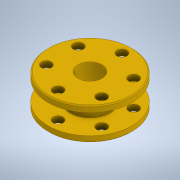
# Autodesk Inventor part: connecting rod hub
Saved by Autodesk Inventor 2020 (Build 240168000, 168)
## iProperties
Created: 2020-08-04
Part Number: connecting rod hub
Material: Generic
Document SubType Name: Modeling
Designer: benny
Density: 1 g/cm^3
Appearance: Gold
Author: benny
Autodesk Inventor part; units mm, degrees
ref_plane "YZ Plane" through (0, 0, 0) normal (1, 0, 0) x (0, 1, 0)
ref_plane "XZ Plane" through (0, 0, 0) normal (0, 1, 0) x (-1, 0, 0)
ref_plane "XY Plane" through (0, 0, 0) normal (0, 0, 1) x (1, 0, 0)
sketch "Sketch1" plane through (0, 0, 0) normal (0, 1, 0) x (-1, 0, 0)
  circle A0 centre (0, 0) radius 10
  dimension "d0" = 20
  constraints: 1 centre point, 1 coincident
  measures "d0" diameter of A0
extrude "Extrusion1" add sketch "Sketch1" along normal mid plane 10
sketch "Sketch2" plane through (0, 5, 0) normal (0, 1, 0) x (1, 0, 0)
  circle A0 centre (0, 0) radius 21
  dimension "d3" = 42
  constraints: 1 centre point, 1 coincident
  measures "d3" diameter of A0
extrude "Extrusion2" add sketch "Sketch2" along normal blind 3
sketch "Sketch3" plane through (0, -5, 0) normal (0, -1, 0) x (1, 0, 0)
  circle A0 centre (0, 0) radius 21
  dimension "d6" = 42
  constraints: 1 centre point, 1 coincident
  measures "d6" diameter of A0
extrude "Extrusion3" add sketch "Sketch3" along normal blind 3
sketch "Sketch4" plane through (0, 8, 0) normal (0, 1, 0) x (1, 0, 0)
  circle A0 centre (0, 0) radius 6
  dimension "d9" = 12
  constraints: 1 centre point, 1 coincident
  measures "d9" diameter of A0
extrude "Extrusion4" cut sketch "Sketch4" against normal blind 16
sketch "Sketch7" plane through (0, 8, 0) normal (0, 1, 0) x (1, 0, 0)
  circle A0 centre (0, -16) radius 2.5
  point P0 (0, 0)
  dimension "d13" = 5
  constraints: 1 centre point
  measures "d13" diameter of A0
extrude "Extrusion5" cut sketch "Sketch7" against normal blind 16
pattern_circular "Circular Pattern1" count 6 over 360 about axis through (0, 5, 0) along (0, 1, 0) of "Extrusion5"
chamfer "Chamfer1" distance 0.5 distance2 0.5 1 edges at (-21, 8, 0) measured on face at (-20.5, 8, 0)
chamfer "Chamfer2" distance 0.5 distance2 0.5 1 edges at (-21, -8, 0) measured on face at (-20.5, -8, 0)
body "Solid1"
